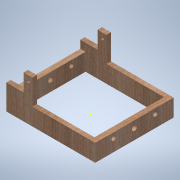
# Autodesk Inventor part: Base
Saved by Autodesk Inventor 2021.3 (Build 253353000, 353)
## iProperties
Created: 2021-06-01
Part Number: Base
Material: Wood (Birch)
Document SubType Name: Modeling
Designer: vivek
Density: 0.55 g/cm^3
Appearance: Birch - Natural Polished
Mass: 886.724 g
Surface Area: 2355.92 cm^2
Volume: 1612.22 cm^3
Author: vivek
Autodesk Inventor part; units mm, degrees
sketch "Sketch1" plane through (0, 0, 0) normal (0, 0, 1) x (1, 0, 0)
  line L0 (150, -133) -> (-150, -133)
  line L1 (-150, -133) -> (-150, 133)
  line L2 (-150, 133) -> (150, 133)
  line L3 (150, 133) -> (150, -133)
  line L4 (0, 0) -> (0, 56.2774)
  line L5 (0, 0) -> (78.3407, 0)
  line L6 (170, -150) -> (-170, -150)
  line L7 (-170, -150) -> (-170, 150)
  line L8 (-170, 150) -> (170, 150)
  line L9 (170, 150) -> (170, -150)
  point P0 (0, 133)
  point P1 (150, 0)
  dimension "d0" = 300
  dimension "d1" = 266
  dimension "d2" = 17
  dimension "d3" = 17
  dimension "d4" = 20
  dimension "d5" = 20
  constraints: 20 end point, 5 parallel, 3 perpendicular, 2 horizontal, 2 midpoint, 2 point on line
  measures "d0" distance of L1.end L2.end
  measures "d1" distance of L0.end L1.end
  measures "d2" distance between parallel lines of L8 L2
  measures "d3" distance between parallel lines of L6 L0
  measures "d4" distance between parallel lines of L7 L1
  measures "d5" distance between parallel lines of L9 L3
extrude "Extrusion1" add sketch "Sketch1" along normal blind 66
sketch "Sketch2" plane through (-170, -150, 0) normal (-1, 0, 0) x (0, 0, 1)
  circle A0 centre (46, 230) radius 8 projected
  circle A1 centre (46, 70) radius 8 projected
  circle A2 centre (46, 230) radius 8
  circle A3 centre (46, 70) radius 8
  circle A4 centre (40, 150) radius 9.5 projected
  circle A5 centre (40, 150) radius 9.5
  point P0 (0, 150)
  constraints: 3 centre point, 3 coincident, 3 concentric
extrude "Extrusion2" cut sketch "Sketch2" against normal through all
sketch "Sketch4" plane through (0, 0, 66) normal (0, 0, 1) x (1, 0, 0)
  line L0 (150, -133) -> (-150, -133) projected
  line L1 (170, 150) -> (-170, 150) projected
  line L2 (-170, 150) -> (-170, -150) projected
  line L3 (-70, -150) -> (-170, -150)
  line L4 (-170, -150) -> (-170, -133)
  line L5 (-170, -133) -> (-70, -133)
  line L6 (-70, -133) -> (-70, -150)
  line L7 (-70, 133) -> (-170, 133)
  line L8 (-170, 133) -> (-170, 150)
  line L9 (-170, 150) -> (-70, 150)
  line L10 (-70, 150) -> (-70, 133)
  point P0 (0, 0)
  dimension "d14" = 100
  dimension "d15" = 17
  dimension "d17" = 100
  dimension "d18" = 17
  constraints: 16 end point, 4 collinear, 4 parallel, 2 horizontal, 2 perpendicular
  measures "d14" distance of L4.end L5.end
  measures "d15" distance of L3.end L4.end
  measures "d17" distance of L8.end L9.end
  measures "d18" distance of L7.end L8.end
extrude "Extrusion3" add sketch "Sketch4" along normal blind 30
ref_plane "Work Plane1" through (-87, -150, 162) normal (0, 0, 1) x (1, 0, 0)
ref_plane "Work Plane2" through (-87, 133, 162) normal (0, 0, 1) x (1, 0, 0)
ref_plane "Work Plane3" through (-87, -150, 162) normal (0, 0, 1) x (1, 0, 0)
sketch "Sketch9" plane through (0, 0, 96) normal (0, 0, 1) x (1, 0, 0)
  line L0 (-70, 133) -> (-70, 150) projected
  line L1 (-70, 150) -> (-170, 150) projected
  line L2 (-104, 133) -> (-104, 150) projected
  line L3 (-70, 133) -> (-104, 133)
  line L4 (-104, 133) -> (-104, 150)
  line L5 (-104, 150) -> (-70, 150)
  line L6 (-70, 150) -> (-70, 133)
  point P0 (0, 0)
  constraints: 8 end point, 2 parallel, 1 horizontal, 1 perpendicular
ref_plane "Work Plane4" through (-157, 133, 162) normal (0, 0, 1) x (1, 0, 0)
extrude "Extrusion8" add sketch "Sketch9" along normal up to surface (66 mm away)
sketch "Sketch10" plane through (0, 0, 96) normal (0, 0, 1) x (1, 0, 0)
  line L0 (-70, -150) -> (-70, -133) projected
  line L1 (-70, -133) -> (-170, -133) projected
  line L2 (-104, -150) -> (-104, -133) projected
  line L3 (-70, -150) -> (-104, -150)
  line L4 (-104, -150) -> (-104, -133)
  line L5 (-104, -133) -> (-70, -133)
  line L6 (-70, -133) -> (-70, -150)
  point P0 (0, 0)
  constraints: 8 end point, 2 parallel, 1 horizontal, 1 perpendicular
ref_plane "Work Plane5" through (-157, -150, 162) normal (0, 0, 1) x (1, 0, 0)
extrude "Extrusion9" add sketch "Sketch10" along normal up to surface (66 mm away)
sketch "Sketch11" plane through (-170, -150, 0) normal (0, -1, 0) x (1, 0, 0)
  circle A0 centre (83, 142) radius 6
  point P0 (170, 0)
  constraints: 1 centre point, 2 other
extrude "Extrusion10" cut sketch "Sketch11" against normal through all
sketch "Sketch12" plane through (0, 0, 0) normal (0, 1, 0) x (-1, 0, 0)
  point P0 (0, 0)
body "Solid1"
